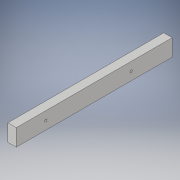
# Autodesk Inventor part: tableSawRunner
Saved by Autodesk Inventor 2019.1 (Build 231200000, 200)
## iProperties
Created: 2018-08-02
Part Number: tableSawRunner
Material: Generic
Document SubType Name: Modeling
Designer: steele
Density: 1 g/cm^3
Appearance: Default
Author: steele
Autodesk Inventor part; units mm, degrees
ref_plane "YZ Plane" through (0, 0, 0) normal (1, 0, 0) x (0, 1, 0)
ref_plane "XZ Plane" through (0, 0, 0) normal (0, 1, 0) x (-1, 0, 0)
ref_plane "XY Plane" through (0, 0, 0) normal (0, 0, 1) x (1, 0, 0)
sketch "Sketch1" plane through (0, 0, 0) normal (0, 1, 0) x (-1, 0, 0)
  line L0 (12.7, 234.95) -> (-12.7, 234.95)
  line L1 (-12.7, 234.95) -> (-12.7, -234.95)
  line L2 (-12.7, -234.95) -> (12.7, -234.95)
  line L3 (12.7, -234.95) -> (12.7, 234.95)
  line L4 (12.7, 234.95) -> (-12.7, -234.95) construction
  line L5 (-12.7, 234.95) -> (12.7, -234.95) construction
  point P0 (0, 0)
  dimension "d0" = 25.4
  dimension "d1" = 469.9
  constraints: 12 end point, 2 midpoint, 2 parallel, 1 horizontal, 1 perpendicular
  measures "d0" distance of L0.start L0.end
  measures "d1" distance of L1.end L0.end
extrude "Extrusion1" add sketch "Sketch1" along normal blind 50.8
sketch "Sketch5" plane through (-12.7, 0, -234.95) normal (-1, 0, 0) x (0, 0, 1)
  line L0 (0, 0) -> (0, 50.8) projected
  circle A0 centre (123.825, 25.4) radius 3.3782
  circle A1 centre (381, 25.4) radius 3.3782
  line L1 (469.9, 0) -> (469.9, 50.8) projected
  point P0 (234.95, 0)
  dimension "d18" = 257.175
  dimension "d20" = 6.7564
  dimension "d21" = 6.7564
  dimension "d24" = 88.9
  constraints: 2 centre point, 2 coincident
  measures "d18" distance of point (381, 25.4) point (123.825, 25.4)
  measures "d20" diameter of A0
  measures "d21" diameter of A1
  measures "d24" distance from line of point (381, 25.4) L1
extrude "Extrusion2" cut sketch "Sketch5" against normal through all
body "Solid1"
